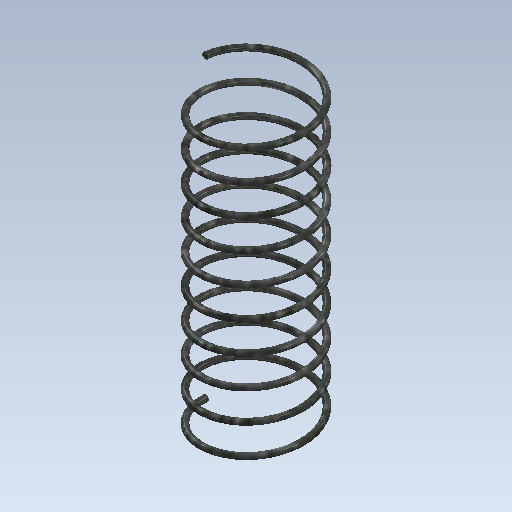
# Autodesk Inventor part: タミヤダンパー部品10
Saved by Autodesk Inventor 2020.2 (Build 242310000, 310)
## iProperties
Created: 2020-02-26
Part Number: タミヤダンパー部品10
Material: 鋼
Document SubType Name: Modeling
Designer: 杉本　賢二郎
Density: 7.85 g/cm^3
Appearance: プレート
Mass: 3.29275 g
Surface Area: 16.8308 cm^2
Volume: 0.419458 cm^3
Author: 杉本　賢二郎
Autodesk Inventor part; units mm, degrees
ref_plane "YZ Plane" through (0, 0, 0) normal (1, 0, 0) x (0, 1, 0)
ref_plane "XZ Plane" through (0, 0, 0) normal (0, 1, 0) x (-1, 0, 0)
ref_plane "XY Plane" through (0, 0, 0) normal (0, 0, 1) x (1, 0, 0)
sketch "スケッチ1" plane through (0, 0, 0) normal (0, 0, 1) x (1, 0, 0)
  circle A0 centre (0, 0) radius 0.5
  line L0 (0, 0) -> (8.5, 0)
  line L1 (8.5, 3) -> (8.5, -3.1992)
  dimension "d0" = 1
  dimension "d1" = 8.5
  dimension "d2" = 3
  constraints: 4 end point, 1 centre point, 1 coincident, 1 horizontal, 1 point on line, 1 vertical
  measures "d0" diameter of A0
  measures "d1" distance of L0.start L0.end
  measures "d2" distance of L0.end L1.start
coil "コイル1" sketch "スケッチ1" operation add axis through (8.5, 3, 0) along (0, -1, 0) pitch 5 turns 10 hand right
